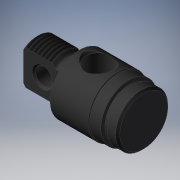
# Autodesk Inventor part: 0.75DXP-C_SRS10
Saved by Autodesk Inventor 2019 (Build 230136000, 136)
## iProperties
Created: 2023-02-15
Part Number: 0.75DXP-C_SRS10
Material: Generic
Catalog Web Link: www.cadenas.de
Description: SR Series Head-Pneumatic Cylinder
Vendor: PARKERHANNIFIN
Document SubType Name: Modeling
Designer: psAdmin
Manufacturer: PARKERHANNIFIN
Mass: 9.27645 g
Surface Area: 34.5606 cm^2
Volume: 9.27645 cm^3
Density: 1 g/cm^3
Appearance: PSOLRGB-175-175-175
Category: PARTsolutions
Company: PARKERHANNIFIN
Title: 0.75DXP-C_SRS10
Author: Cadenas PARTsolutions
Comments: Pneumatic Cylinder
PSOL_IDENT_0: {$CADENAS_DATA/23d-libs/parkerpdn/actuators_cylinders/pneumatic_cylinders/sr_series/parts/sr_head_ca
PSOL_IDENT_1: p.prj},209 {VTYP=3D},{NB=0.75DXP-C_SRS10},{LINA=0.75DXP-C_SRS10},{NN=SR Series Head},{DATE=26.07.202
PSOL_IDENT_2: 1 05:25:39},{GEOMDATE=25.09.2019 05:53:45},{VERSION=},{LINEID=40},{WBVAR=MNT,USE,CUH,SPEC,PL,SER,NL,
PSOL_IDENT_3: RRPT},{WBNUMERIC=}  {NB=0.75DXP-C_SRS10},{LINA=0.75DXP-C_SRS10},{KT=DUMMY},{PN=0.75DXP-C_SR},{BORE=0
PSOL_IDENT_4: .7500},{BORECON=0.7500},{MNT=DXP},{MNTALG= 'N' , 'N - Nose Mount, Spring Return' , 'NR' , 'NR - Nose
PSOL_IDENT_5: Mount, Spring Return, Hex Rod (non-rotating)' , 'NRP' , 'NRP - Pivot and Nose Mount, Spring Return,
PSOL_IDENT_6: Hex Rod (non-rotating)' , 'P' , 'P - Pivot Mount, Spring Return' , 'R' , 'R - Nose Mount, Spring Ex
PSOL_IDENT_7: tended' , 'RP' , 'RP - Pivot and Nose Mount, Spring Extend' , 'D' , 'D - Nose Mount, Double Acting','
PSOL_IDENT_8: DP' , 'DP - Pivot and Nose Mount, Double Acting, Pivot Pin' , 'DXP' , 'DXP - Pivot and Nose Mount, D
PSOL_IDENT_9: ouble Acting, No Pivot Pin' , 'DX' , 'DX - Threaded Both End, Double Acting' ,  'A' , 'A - Nose Moun
PSOL_IDENT_10: t, Spring Return, Head Adjustable Stroke' , 'RA' , 'RA - Nose Mount, Spring Extend, Cap Adjustable S
PSOL_IDENT_11: troke' , 'AP' , 'AP - Pivot Mount, Spring Return, Head Adjustable Stroke' , 'AR' , 'AR - Air Reservo
PSOL_IDENT_12: irs' , 'BRN' , 'BRN - Rear Block Mount, Single Acting' , 'BRR' , 'BRR - Rear Block Mount, Single Act
PSOL_IDENT_13: ing, Spring Return' , 'BFD' , 'BFD - Front Block Mount, Double Acting' , 'BRD' , 'BRD - Rear Block M
PSOL_IDENT_14: ount, Double Acting' , 'BFN' , 'BFN - Front Block Mount, Single Acting, Spring Return' , 'BFR' , 'BF
PSOL_IDENT_15: R - Front Block Mount, Single Acting, Spring Extend' , 'TRN' , 'TRN - Rear Trunnion Mount, Single Ac
PSOL_IDENT_16: ting, Spring Return' , 'TRR' , 'TRR - Rear Trunnion Mount, Single Acting, Spring Extend' , 'TFD' , '
PSOL_IDENT_17: TFD - Front Trunnion Mount, Double Acting' , 'TRD' , 'TRD - Rear Trunnion Mount, Double Acting' , 'T
PSOL_IDENT_18: FN' , 'TFN - Front Trunnion Mount, Single Acting, Spring Return' , 'TFR' , 'TFR - Front Trunnion Mou
PSOL_IDENT_19: nt, Single Acting, Spring Extend' },{USE=C},{USEALG=  'H', 'Head', 'C', 'Cap' },{CUH=},{CUHALG= '' ,
PSOL_IDENT_20: 'No Cushion' , 'C' , 'C - Cushion' },{SPEC=S},{PL=1},{THD=0.6250},{THD1=0.5000},{THD2=0.5000},{THD3=
PSOL_IDENT_21: 0.6250},{TAB=UNF},{L=1.56200},{OD=0.85500},{SQ=0.00000},{SQW=0.00000},{THDLEN=0.42200},{L1=0.93300},
PSOL_IDENT_22: {L2=0.38000},{L3=0.21500},{L31=0.18800},{L4=0.03600},{D1=0.70100},{D2=0.75800},{D3=0.00000},{D4=0.81
PSOL_IDENT_23: 500},{C1=0.03000},{CC=0.25000},{PD=0.44000},{PLHELP=1},{ROT=-90},{EETHD=0.40500},{EETHD1=0.40500},{E
PSOL_IDENT_24: ETAB=NPTF},{CBOREDEP=0.00000},{CBOREDIA=0.00000},{HEX=0.00000},{HEXDEP=0.00000},{XW=0.00000},{XD=0.0
PSOL_IDENT_25: 0000},{TD=0.50000},{TL=0.37500},{TRDIS=0.37000},{TRDIS1=0.35000},{TRDIS2=0.37000},{DA=0.00000},{DADE
PSOL_IDENT_26: P=0.00000},{DB=0.00000},{CF=0.00000},{CP=0.00000},{HP=0.62500},{FH=0.37500},{BC=1.00000},{S=0.19000}
PSOL_IDENT_27: ,{SDEP=0.34400},{STAB=UNF},{ASTHD=0.43750},{SO=0.25000},{SODEP=0.50000},{SC=0.33300},{SCDEP=0.20800}
PSOL_IDENT_28: ,{CL1=0.08200},{CL2=0.12500},{CD1=0.62200},{CD2=0.53700},{CR1=0.03000},{CUX=0.62500},{CUY=0.25900},{
PSOL_IDENT_29: CUD1=0.22800},{CUD2=0.16100},{FOD=0.34300},{CUD2DEP=0.15600},{CUTHD=3.000},{PCUT=0.37000},{PCUT1=0.3
PSOL_IDENT_30: 7000},{PCUT2=0.00000},{PCUTDEP=0.00800},{PDIA=0.25150},{PDIA1=0.25150},{PDIA2=0.25000},{PDIA3=0.3140
PSOL_IDENT_31: 0},{PDIS=1.07000},{PDIS1=1.07000},{WC=0.00000},{WCDEP=0.18800},{NOTHD=0},{LENGTH=1.34700},{NUTCON=0.
PSOL_IDENT_32: 625},{OLEN=1.56200},{BUSH=0},{SER=SR},{PLCALG='None','None','1','Port Position 1 Cap End','2','Port
PSOL_IDENT_33: Position 2 Cap End','3','Port Position 3 Cap End','4','Port Position 4 Cap End','5','Port On Face'},
PSOL_IDENT_34: {PLHELP1=1},{NL=},{ROTCUH=0.000},{NLALG='','N/A'},{RRPT=0},{RRPTALG='0','No','1','Yes'}
NB: 0.75DXP-C_SRS10
NN: SR Series Head
NT: Pneumatic Cylinder
NBSYN: $PN.$SPEC.$PL.$NL.$RRPT.
LINA: 0.75DXP-C_SRS10
CATALOG: Parker Pneumatic Division
BORE: 0.75
BORECON: 0.7500
MNT: DXP - Pivot and Nose Mount, Double Acting, No Pivot Pin
USE: Cap
CUH: No Cushion
SPEC: Special Modifications
PL: Port Position 1 Cap End
THD1: 0.5
THD2: 0.5
THD3: 0.625
TAB: UNF
L31: 0.188
L4: 0.036
D1: 0.701
D2: 0.758
C1: 0.03
CC: 0.25
EETHD1: 0.405
EETAB: NPTF
TD: 0.5
TL: 0.375
TRDIS1: 0.35
TRDIS2: 0.37
DA: 0
DADEP: 0
DB: 0
CF: 0
CP: 0
HP: 0.625
FH: 0.375
BC: 1
S: 0.19
SDEP: 0.344
STAB: UNF
ASTHD: 0.4375
SO: 0.25
SODEP: 0.5
SC: 0.333
SCDEP: 0.208
CL1: 0.082
CR1: 0.03
CUX: 0.625
CUY: 0.259
CUD1: 0.228
CUD2: 0.161
FOD: 0.343
CUD2DEP: 0.156
CUTHD: 3
PCUT1: 0.37
PCUT2: 0
PCUTDEP: 0.008
PDIA1: 0.2515
PDIA2: 0.25
PDIA3: 0.314
PDIS1: 1.07
WCDEP: 0.188
SER: SR
NL: N/A
RRPT: No
SUPPLIER: PARKERHANNIFIN
ARTICLENO: 0.75DXP-C_SRS10
BOMINFO: 0.75DXP-C_SRS10
CREATOR: CADENAS GmbH
Autodesk Inventor part; units mm, degrees
sketch "Sketch_1" plane through (0, 0, 0) normal (0, 0, 1) x (1, 0, 0)
  line L0 (14.0462, 0) -> (0, 0)
  line L1 (0, 0) -> (0, 10.8585)
  line L2 (0, 10.8585) -> (14.0462, 10.8585)
  line L3 (14.0462, 10.8585) -> (14.0462, 0)
  line L4 (14.0462, 0) -> (0, 0)
  constraints: 10 end point
revolve "Revolution1" add sketch "Sketch_1" angle 360 about axis through (14.0462, 0, 0) along (1, 0, 0)
sketch "Sketch_2" plane through (0, 0, 0) normal (0, 0, 1) x (1, 0, 0)
  line L0 (0, 0) -> (-15.9766, 0)
  line L1 (-15.9766, 0) -> (-15.9766, 7.098)
  line L2 (-15.9766, 7.098) -> (-15.1371, 7.9375)
  line L3 (-15.1371, 7.9375) -> (0, 7.9375)
  line L4 (0, 7.9375) -> (0, 0)
  line L5 (0, 0) -> (-15.9766, 0)
  constraints: 12 end point
revolve "Revolution2" add sketch "Sketch_2" angle 360 about axis through (0, 0, 0) along (1, 0, 0)
thread "Thread1" size "5/8-18 UNF" class "2A" standard "ANSI Unified Screw Threads" length 9.8793
sketch "Sketch_6" plane through (0, 0, 0) normal (0, 0, 1) x (1, 0, 0)
  line L0 (23.6982, 0) -> (14.0462, 0)
  line L1 (14.0462, 0) -> (14.0462, 10.3505)
  line L2 (14.0462, 10.3505) -> (18.2372, 10.3505)
  line L3 (18.2372, 10.3505) -> (18.2372, 8.9027)
  line L4 (18.2372, 8.9027) -> (19.1516, 8.9027)
  line L5 (19.1516, 8.9027) -> (19.8755, 9.6266)
  line L6 (19.8755, 9.6266) -> (22.9362, 9.6266)
  line L7 (22.9362, 9.6266) -> (23.6982, 8.8646)
  line L8 (23.6982, 8.8646) -> (23.6982, 0)
  line L9 (23.6982, 0) -> (14.0462, 0)
  constraints: 20 end point
revolve "Revolution3" add sketch "Sketch_6" angle 360 about axis through (23.6982, 0, 0) along (1, 0, 0)
sketch "Sketch_8" plane through (7.0612, 0, 0) normal (0, 0, 1) x (0, -1, 0)
  line L0 (0, 0) -> (-11.7085, 0)
  line L1 (-11.7085, 0) -> (-11.7085, 6.4547)
  line L2 (-11.7085, 6.4547) -> (-10.0692, 4.8153)
  line L3 (-10.0692, 4.8153) -> (0, 4.501)
  line L4 (0, 4.501) -> (0, 0)
  line L5 (0, 0) -> (-11.7085, 0)
  constraints: 12 end point
revolve "Revolution4" cut sketch "Sketch_8" angle 360 about axis through (7.0612, 0, 0) along (0, -1, 0)
sketch "Sketch_29" plane through (0, 0, 0) normal (0, 0, 1) x (1, 0, 0)
  line L0 (0, 0) -> (-5.2578, 0)
  line L1 (-5.2578, 9.8994) -> (-5.2578, 7.9375)
  line L2 (-5.2578, 7.9375) -> (-4.3634, 7.0431)
  arc A0 (-4.3634, 7.0431) -> (-3.8246, 6.8199) centre (-3.8246, 7.5819) ccw
  line L3 (-3.8246, 6.8199) -> (-2.7567, 6.8199)
  arc A1 (-2.7567, 6.8199) -> (-2.0828, 7.2263) centre (-2.7567, 7.5819) ccw
  line L4 (-2.0828, 7.2263) -> (-2.0828, 7.8994)
  line L5 (-2.0828, 7.8994) -> (0, 7.8994)
  line L6 (0, 7.8994) -> (0, 9.8994)
  line L7 (0, 9.8994) -> (-5.2578, 9.8994)
  constraints: 16 end point, 4 point on circle, 2 centre point
revolve "Revolution5" cut sketch "Sketch_29" angle 360 about axis through (0, 0, 0) along (1, 0, 0)
sketch "Sketch_38" plane through (-0.2032, 0, 0) normal (1, 0, 0) x (0, 0, -1)
  line L0 (-10.8585, -10.8585) -> (10.8585, -10.8585)
  line L1 (10.8585, -10.8585) -> (10.8585, 10.8585)
  line L2 (10.8585, 10.8585) -> (-10.8585, 10.8585)
  line L3 (-10.8585, 10.8585) -> (-10.8585, -10.8585)
  line L4 (-4.699, -8.7312) -> (4.699, -8.7312)
  line L5 (4.699, -8.7312) -> (4.699, 8.7312)
  line L6 (4.699, 8.7312) -> (-4.699, 8.7312)
  line L7 (-4.699, 8.7312) -> (-4.699, -8.7312)
  constraints: 16 end point
extrude "Extrusion1" cut sketch "Sketch_38" against normal blind 15.9766
sketch "Sketch_36" plane through (0, 0, 0) normal (0, 1, 0) x (-1, 0, 0)
  line L0 (8.9408, 4.699) -> (8.9408, -4.699)
  line L1 (8.9408, -4.699) -> (5.1079, -4.699)
  line L2 (5.1079, -4.699) -> (5.7467, -4.0602)
  line L3 (5.7467, -4.0602) -> (5.7467, 4.0602)
  line L4 (5.7467, 4.0602) -> (5.1079, 4.699)
  line L5 (5.1079, 4.699) -> (8.9408, 4.699)
  line L6 (8.9408, 4.699) -> (8.9408, -4.699)
  constraints: 14 end point
revolve "Revolution6" cut sketch "Sketch_36" angle 360 about axis through (-8.9408, 0, 4.699) along (0, 0, 1)
ref_plane "b1_XY" through (0, 7.8994, 0) normal (1, 0, 0) x (0, 0, -1)
ref_plane "b1_YZ" through (0, 7.8994, 0) normal (0, 0, -1) x (0, 1, 0)
ref_plane "b1_ZX" through (0, 7.8994, 0) normal (0, 1, 0) x (1, 0, 0)
ref_plane "b2_XY" through (0, -7.8994, 0) normal (1, 0, 0) x (0, 0, -1)
ref_plane "b2_YZ" through (0, -7.8994, 0) normal (0, 0, -1) x (0, 1, 0)
ref_plane "b2_ZX" through (0, -7.8994, 0) normal (0, 1, 0) x (1, 0, 0)
ref_plane "cl1_XY" through (0, 0, 0) normal (0, 0, 1) x (1, 0, 0)
ref_plane "cl1_YZ" through (0, 0, 0) normal (1, 0, 0) x (0, 1, 0)
ref_plane "cl1_ZX" through (0, 0, 0) normal (0, 1, 0) x (0, 0, 1)
ref_plane "cl2_XY" through (-2.0828, 0, 0) normal (0, 0, 1) x (1, 0, 0)
ref_plane "cl2_YZ" through (-2.0828, 0, 0) normal (1, 0, 0) x (0, 1, 0)
ref_plane "cl2_ZX" through (-2.0828, 0, 0) normal (0, 1, 0) x (0, 0, 1)
ref_plane "ecut1_XY" through (-0.2032, 0, 4.699) normal (1, 0, 0) x (0, 0, -1)
ref_plane "ecut1_YZ" through (-0.2032, 0, 4.699) normal (0, 0, -1) x (0, 1, 0)
ref_plane "ecut1_ZX" through (-0.2032, 0, 4.699) normal (0, 1, 0) x (1, 0, 0)
ref_plane "ecut2_XY" through (-0.2032, 0, -4.699) normal (1, 0, 0) x (0, 0, -1)
ref_plane "ecut2_YZ" through (-0.2032, 0, -4.699) normal (0, 0, -1) x (0, 1, 0)
ref_plane "ecut2_ZX" through (-0.2032, 0, -4.699) normal (0, 1, 0) x (1, 0, 0)
ref_plane "ee_XY" through (7.0612, 10.8585, 0) normal (1, 0, 0) x (0, -1, 0)
ref_plane "ee_YZ" through (7.0612, 10.8585, 0) normal (0, -1, 0) x (0, 0, -1)
ref_plane "ee_ZX" through (7.0612, 10.8585, 0) normal (0, 0, -1) x (1, 0, 0)
ref_plane "od1_XY" through (0, 0, 10.8585) normal (1, 0, 0) x (0, 0, -1)
ref_plane "od1_YZ" through (0, 0, 10.8585) normal (0, 0, -1) x (0, 1, 0)
ref_plane "od1_ZX" through (0, 0, 10.8585) normal (0, 1, 0) x (1, 0, 0)
ref_plane "od2_XY" through (0, 0, -10.8585) normal (1, 0, 0) x (0, 0, -1)
ref_plane "od2_YZ" through (0, 0, -10.8585) normal (0, 0, -1) x (0, 1, 0)
ref_plane "od2_ZX" through (0, 0, -10.8585) normal (0, 1, 0) x (1, 0, 0)
ref_plane "od3_XY" through (0, 10.8585, 0) normal (1, 0, 0) x (0, 0, -1)
ref_plane "od3_YZ" through (0, 10.8585, 0) normal (0, 0, -1) x (0, 1, 0)
ref_plane "od3_ZX" through (0, 10.8585, 0) normal (0, 1, 0) x (1, 0, 0)
ref_plane "od4_XY" through (0, -10.8585, 0) normal (1, 0, 0) x (0, 0, -1)
ref_plane "od4_YZ" through (0, -10.8585, 0) normal (0, 0, -1) x (0, 1, 0)
ref_plane "od4_ZX" through (0, -10.8585, 0) normal (0, 1, 0) x (1, 0, 0)
ref_plane "to_body_XY" through (18.2372, 0, 0) normal (1, 0, 0) x (0, 0, -1)
ref_plane "to_body_YZ" through (18.2372, 0, 0) normal (0, 0, -1) x (0, 1, 0)
ref_plane "to_body_ZX" through (18.2372, 0, 0) normal (0, 1, 0) x (1, 0, 0)
ref_plane "to_dummy_XY" through (0, 0, 0) normal (1, 0, 0) x (0, 0, -1)
ref_plane "to_dummy_YZ" through (0, 0, 0) normal (0, 0, -1) x (0, 1, 0)
ref_plane "to_dummy_ZX" through (0, 0, 0) normal (0, 1, 0) x (1, 0, 0)
ref_plane "to_nut_XY" through (-15.9766, 0, 0) normal (1, 0, 0) x (0, 0, -1)
ref_plane "to_nut_YZ" through (-15.9766, 0, 0) normal (0, 0, -1) x (0, 1, 0)
ref_plane "to_nut_ZX" through (-15.9766, 0, 0) normal (0, 1, 0) x (1, 0, 0)
ref_plane "to_pin_XY" through (-8.9408, 0, 0) normal (0, 0, 1) x (1, 0, 0)
ref_plane "to_pin_YZ" through (-8.9408, 0, 0) normal (1, 0, 0) x (0, 1, 0)
ref_plane "to_pin_ZX" through (-8.9408, 0, 0) normal (0, 1, 0) x (0, 0, 1)
ref_plane "to_stroke_adjuster_XY" through (23.6982, 0, 0) normal (1, 0, 0) x (0, 0, -1)
ref_plane "to_stroke_adjuster_YZ" through (23.6982, 0, 0) normal (0, 0, -1) x (0, 1, 0)
ref_plane "to_stroke_adjuster_ZX" through (23.6982, 0, 0) normal (0, 1, 0) x (1, 0, 0)
ref_plane "z1_XY" through (-8.9408, 3.194, 0) normal (0, 0, 1) x (1, 0, 0)
ref_plane "z1_YZ" through (-8.9408, 3.194, 0) normal (1, 0, 0) x (0, 1, 0)
ref_plane "z1_ZX" through (-8.9408, 3.194, 0) normal (0, 1, 0) x (0, 0, 1)
ref_plane "z2_XY" through (-8.9408, -3.194, 0) normal (0, 0, 1) x (1, 0, 0)
ref_plane "z2_YZ" through (-8.9408, -3.194, 0) normal (1, 0, 0) x (0, 1, 0)
ref_plane "z2_ZX" through (-8.9408, -3.194, 0) normal (0, 1, 0) x (0, 0, 1)
body "Solid1"
